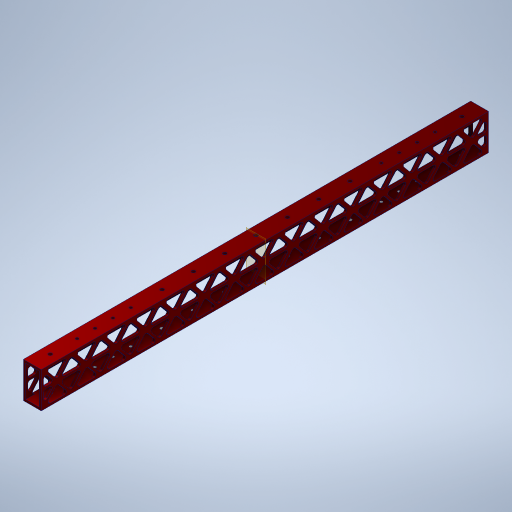
# Autodesk Inventor part: Drivetrain-Front-Back-Extrusions
Saved by Autodesk Inventor 2024.2 (Build 282272000, 272)
## iProperties
Created: 2024-01-04
Part Number: Drivetrain-Front-Back-Extrusions
Material: Aluminum 6061
Document SubType Name: Modeling
Designer: rohan
Density: 2.7 g/cm^3
Appearance: Aluminum - Flat
Author: rohan
Autodesk Inventor part; units mm, degrees
ref_plane "YZ Plane" through (0, 0, 0) normal (1, 0, 0) x (0, 1, 0)
ref_plane "XZ Plane" through (0, 0, 0) normal (0, 1, 0) x (-1, 0, 0)
ref_plane "XY Plane" through (0, 0, 0) normal (0, 0, 1) x (1, 0, 0)
sketch "Sketch1" plane through (0, 0, 0) normal (0, 0, 1) x (1, 0, 0)
  line L0 (-12.7, -25.4) -> (12.7, -25.4)
  line L1 (12.7, -25.4) -> (12.7, 25.4)
  line L2 (12.7, 25.4) -> (-12.7, 25.4)
  line L3 (-12.7, 25.4) -> (-12.7, -25.4)
  line L4 (-12.7, -25.4) -> (12.7, 25.4) construction
  line L5 (12.7, -25.4) -> (-12.7, 25.4) construction
  line L6 (-9.525, -22.225) -> (9.525, -22.225)
  line L7 (9.525, -22.225) -> (9.525, 22.225)
  line L8 (9.525, 22.225) -> (-9.525, 22.225)
  line L9 (-9.525, 22.225) -> (-9.525, -22.225)
  point P0 (0, 0)
  dimension "d0" = 25.4
  dimension "d1" = 50.8
  dimension "d2" = 3.175
  constraints: 20 end point, 4 parallel, 2 midpoint, 2 perpendicular, 1 horizontal, 3 other
  measures "d0" distance of L2.end L1.end
  measures "d1" distance of L1.end L0.end
  measures "d2" distance between parallel lines of L3 L9
extrude "Extrusion1" add sketch "Sketch1" along normal blind 635
sketch "Sketch2" plane through (-12.7, 25.4, 0) normal (0, 1, 0) x (1, 0, 0)
  circle A0 centre (12.7, -25.4) radius 2.5527
  circle A1 centre (12.7, -63.5) radius 2.0193
  line L0 (25.4, 0) -> (25.4, -635) projected
  circle A2 centre (12.7, -88.9) radius 2.0193
  circle A3 centre (12.7, -114.3) radius 2.0193
  circle A4 centre (12.7, -139.7) radius 2.0193
  point P0 (12.7, 0)
  dimension "d5" = 5.1054
  dimension "d6" = 25.4
  dimension "d7" = 4.0386
  dimension "d8" = 63.5
  dimension "d11" = 25.4
  constraints: 5 centre point, 1 vertical, 6 other
  measures "d5" diameter of A0
  measures "d6" distance of A0.centre point (12.7, 0)
  measures "d7" diameter of A1
  measures "d8" distance of A1.centre point (12.7, 0)
  measures "d11" distance of A1.centre A2.centre
extrude "Extrusion2" cut sketch "Sketch2" against normal blind 111.125
ref_plane "Work Plane1" through (0, 0, 317.5) normal (0, 0, 1) x (1, 0, 0)
mirror "Mirror1" about plane through (0, 0, 317.5) normal (0, 0, 1) of "Extrusion2"
sketch "Sketch5" plane through (12.7, -25.4, 0) normal (1, 0, 0) x (0, 0, -1)
  line L0 (-635, 0) -> (-635, 50.8) projected
  line L1 (-635, 25.4) -> (0, 25.4)
  line L2 (0, 50.8) -> (-635, 50.8) projected
  line L3 (-317.5, 50.8) -> (-317.5, 0)
  line L4 (-631.825, 30.1625) -> (-631.825, 37.2672)
  line L5 (-628.65, 26.9875) -> (-622.6851, 26.9875)
  line L6 (-620.2534, 32.204) -> (-626.2184, 39.3087)
  arc A0 (-626.2184, 39.3087) -> (-631.825, 37.2672) centre (-628.65, 37.2672) ccw
  arc A1 (-631.825, 30.1625) -> (-628.65, 26.9875) centre (-628.65, 30.1625) ccw
  arc A2 (-622.6851, 26.9875) -> (-620.2534, 32.204) centre (-622.6851, 30.1625) ccw
  line L7 (-631.825, 20.6375) -> (-631.825, 13.5328)
  line L8 (-628.65, 23.8125) -> (-622.6851, 23.8125)
  line L9 (-620.2534, 18.596) -> (-626.2184, 11.4913)
  arc A3 (-631.825, 13.5328) -> (-626.2184, 11.4913) centre (-628.65, 13.5328) ccw
  arc A4 (-628.65, 23.8125) -> (-631.825, 20.6375) centre (-628.65, 20.6375) ccw
  arc A5 (-620.2534, 18.596) -> (-622.6851, 23.8125) centre (-622.6851, 20.6375) ccw
  line L10 (-626.2184, 11.4913) -> (-620.2534, 18.596)
  line L11 (-617.8218, 16.5545) -> (-623.7867, 9.4497)
  line L12 (-623.7867, 9.4497) -> (-624.6752, 8.3915)
  line L13 (-622.2436, 3.175) -> (-602.7132, 3.175)
  line L14 (-600.2863, 8.3971) -> (-610.0741, 20.0012)
  line L15 (-624.6752, 8.3915) -> (-614.9327, 19.9956)
  arc A6 (-624.6752, 8.3915) -> (-622.2436, 3.175) centre (-622.2436, 6.35) ccw
  arc A7 (-602.7132, 3.175) -> (-600.2863, 8.3971) centre (-602.7132, 6.35) ccw
  arc A8 (-610.0741, 20.0012) -> (-614.9327, 19.9956) centre (-612.5011, 17.9541) ccw
  line L16 (-608.3475, 17.9541) -> (-602.1017, 10.5494)
  line L17 (-604.7305, 18.5904) -> (-599.6748, 12.5965)
  line L18 (-602.3036, 23.8125) -> (-582.8708, 23.8125)
  line L19 (-599.6748, 12.5965) -> (-604.7305, 18.5904)
  line L20 (-604.7305, 18.5904) -> (-595.0141, 7.0711)
  line L21 (-585.4997, 12.5965) -> (-580.4439, 18.5904)
  line L22 (-580.4439, 18.5904) -> (-590.1603, 7.0711)
  arc A9 (-595.0141, 7.0711) -> (-590.1603, 7.0711) centre (-592.5872, 9.1182) ccw
  arc A10 (-602.3036, 23.8125) -> (-604.7305, 18.5904) centre (-602.3036, 20.6375) ccw
  arc A11 (-580.4439, 18.5904) -> (-582.8708, 23.8125) centre (-582.8708, 20.6375) ccw
  line L23 (-623.7867, 41.3503) -> (-615.5957, 41.3503) construction
  line L24 (-622.2436, 47.625) -> (-602.7132, 47.625)
  line L25 (-600.2863, 42.4029) -> (-610.0741, 30.7988)
  line L26 (-624.6752, 42.4085) -> (-614.9327, 30.8044)
  arc A12 (-622.2436, 47.625) -> (-624.6752, 42.4085) centre (-622.2436, 44.45) ccw
  arc A13 (-600.2863, 42.4029) -> (-602.7132, 47.625) centre (-602.7132, 44.45) ccw
  arc A14 (-614.9327, 30.8044) -> (-610.0741, 30.7988) centre (-612.5011, 32.8459) ccw
  line L27 (-608.3475, 32.8459) -> (-602.1017, 40.2506)
  line L28 (-604.7305, 32.2096) -> (-599.6748, 38.2035)
  line L29 (-602.3036, 26.9875) -> (-582.8708, 26.9875)
  line L30 (-599.6748, 38.2035) -> (-604.7305, 32.2096)
  line L31 (-604.7305, 32.2096) -> (-595.0141, 43.7289)
  line L32 (-585.4997, 38.2035) -> (-580.4439, 32.2096)
  line L33 (-580.4439, 32.2096) -> (-590.1603, 43.7289)
  arc A15 (-590.1603, 43.7289) -> (-595.0141, 43.7289) centre (-592.5872, 41.6818) ccw
  arc A16 (-604.7305, 32.2096) -> (-602.3036, 26.9875) centre (-602.3036, 30.1625) ccw
  arc A17 (-582.8708, 26.9875) -> (-580.4439, 32.2096) centre (-582.8708, 30.1625) ccw
  line L34 (-3.175, 30.1625) -> (-3.175, 37.2672)
  line L35 (-6.35, 26.9875) -> (-12.3149, 26.9875)
  line L36 (-14.7466, 32.204) -> (-8.7816, 39.3087)
  arc A18 (-3.175, 37.2672) -> (-8.7816, 39.3087) centre (-6.35, 37.2672) ccw
  arc A19 (-6.35, 26.9875) -> (-3.175, 30.1625) centre (-6.35, 30.1625) ccw
  arc A20 (-14.7466, 32.204) -> (-12.3149, 26.9875) centre (-12.3149, 30.1625) ccw
  arc A21 (-8.7816, 11.4913) -> (-3.175, 13.5328) centre (-6.35, 13.5328) ccw
  line L37 (-3.175, 20.6375) -> (-3.175, 13.5328)
  line L38 (-14.7466, 18.596) -> (-8.7816, 11.4913)
  arc A22 (-3.175, 20.6375) -> (-6.35, 23.8125) centre (-6.35, 20.6375) ccw
  line L39 (-6.35, 23.8125) -> (-12.3149, 23.8125)
  arc A23 (-12.3149, 23.8125) -> (-14.7466, 18.596) centre (-12.3149, 20.6375) ccw
  line L40 (-8.7816, 11.4913) -> (-14.7466, 18.596)
  line L41 (-17.1782, 16.5545) -> (-11.2133, 9.4497)
  line L42 (-11.2133, 9.4497) -> (-10.3248, 8.3915)
  line L43 (-12.7564, 3.175) -> (-32.2868, 3.175)
  line L44 (-34.7137, 8.3971) -> (-24.9259, 20.0012)
  line L45 (-10.3248, 8.3915) -> (-20.0673, 19.9956)
  arc A24 (-12.7564, 3.175) -> (-10.3248, 8.3915) centre (-12.7564, 6.35) ccw
  arc A25 (-34.7137, 8.3971) -> (-32.2868, 3.175) centre (-32.2868, 6.35) ccw
  arc A26 (-20.0673, 19.9956) -> (-24.9259, 20.0012) centre (-22.4989, 17.9541) ccw
  arc A27 (-32.2868, 47.625) -> (-34.7137, 42.4029) centre (-32.2868, 44.45) ccw
  arc A28 (-24.9259, 30.7988) -> (-20.0673, 30.8044) centre (-22.4989, 32.8459) ccw
  line L46 (-12.7564, 47.625) -> (-32.2868, 47.625)
  line L47 (-34.7137, 42.4029) -> (-24.9259, 30.7988)
  line L48 (-11.2133, 41.3503) -> (-19.4043, 41.3503) construction
  line L49 (-10.3248, 42.4085) -> (-20.0673, 30.8044)
  arc A29 (-10.3248, 42.4085) -> (-12.7564, 47.625) centre (-12.7564, 44.45) ccw
  arc A30 (-538.4069, 18.5904) -> (-540.8338, 23.8125) centre (-540.8338, 20.6375) ccw
  arc A31 (-540.8338, 26.9875) -> (-538.4069, 32.2096) centre (-540.8338, 30.1625) ccw
  line L50 (-543.4627, 38.2035) -> (-538.4069, 32.2096)
  line L51 (-538.4069, 32.2096) -> (-548.1233, 43.7289)
  line L52 (-560.2666, 23.8125) -> (-540.8338, 23.8125)
  arc A32 (-558.2493, 42.4029) -> (-560.6762, 47.625) centre (-560.6762, 44.45) ccw
  line L53 (-562.6935, 32.2096) -> (-552.9771, 43.7289)
  line L54 (-562.6935, 32.2096) -> (-557.6378, 38.2035)
  line L55 (-557.6378, 38.2035) -> (-562.6935, 32.2096)
  line L56 (-592.963, 25.4) -> (42.037, 25.4)
  line L57 (-560.2666, 26.9875) -> (-540.8338, 26.9875)
  arc A33 (-568.0371, 20.0012) -> (-572.8957, 19.9956) centre (-570.4641, 17.9541) ccw
  arc A34 (-560.2666, 23.8125) -> (-562.6935, 18.5904) centre (-560.2666, 20.6375) ccw
  line L58 (-575.7848, 16.5545) -> (-581.7497, 9.4497)
  line L59 (-580.2066, 3.175) -> (-560.6762, 3.175)
  line L60 (-582.6382, 8.3915) -> (-572.8957, 19.9956)
  line L61 (-558.2493, 8.3971) -> (-568.0371, 20.0012)
  arc A35 (-560.6762, 3.175) -> (-558.2493, 8.3971) centre (-560.6762, 6.35) ccw
  line L62 (-566.3105, 17.9541) -> (-560.0647, 10.5494)
  line L63 (-562.6935, 18.5904) -> (-557.6378, 12.5965)
  line L64 (-557.6378, 12.5965) -> (-562.6935, 18.5904)
  line L65 (-562.6935, 18.5904) -> (-552.9771, 7.0711)
  line L66 (-543.4627, 12.5965) -> (-538.4069, 18.5904)
  line L67 (-538.4069, 18.5904) -> (-548.1233, 7.0711)
  arc A36 (-552.9771, 7.0711) -> (-548.1233, 7.0711) centre (-550.5502, 9.1182) ccw
  arc A37 (-548.1233, 43.7289) -> (-552.9771, 43.7289) centre (-550.5502, 41.6818) ccw
  line L68 (-582.6382, 42.4085) -> (-572.8957, 30.8044)
  line L69 (-581.7497, 41.3503) -> (-573.5587, 41.3503) construction
  line L70 (-580.2066, 47.625) -> (-560.6762, 47.625)
  arc A38 (-572.8957, 30.8044) -> (-568.0371, 30.7988) centre (-570.4641, 32.8459) ccw
  line L71 (-566.3105, 32.8459) -> (-560.0647, 40.2506)
  arc A39 (-562.6935, 32.2096) -> (-560.2666, 26.9875) centre (-560.2666, 30.1625) ccw
  line L72 (-558.2493, 42.4029) -> (-568.0371, 30.7988)
  arc A40 (-582.6382, 8.3915) -> (-580.2066, 3.175) centre (-580.2066, 6.35) ccw
  arc A41 (-580.2066, 47.625) -> (-582.6382, 42.4085) centre (-580.2066, 44.45) ccw
  arc A42 (-496.3699, 18.5904) -> (-498.7968, 23.8125) centre (-498.7968, 20.6375) ccw
  arc A43 (-498.7968, 26.9875) -> (-496.3699, 32.2096) centre (-498.7968, 30.1625) ccw
  line L73 (-501.4257, 38.2035) -> (-496.3699, 32.2096)
  line L74 (-496.3699, 32.2096) -> (-506.0863, 43.7289)
  line L75 (-518.2296, 23.8125) -> (-498.7968, 23.8125)
  arc A44 (-516.2123, 42.4029) -> (-518.6392, 47.625) centre (-518.6392, 44.45) ccw
  line L76 (-520.6565, 32.2096) -> (-510.9401, 43.7289)
  line L77 (-520.6565, 32.2096) -> (-515.6008, 38.2035)
  line L78 (-515.6008, 38.2035) -> (-520.6565, 32.2096)
  line L79 (-550.926, 25.4) -> (84.074, 25.4)
  line L80 (-518.2296, 26.9875) -> (-498.7968, 26.9875)
  arc A45 (-526.0001, 20.0012) -> (-530.8587, 19.9956) centre (-528.4271, 17.9541) ccw
  arc A46 (-518.2296, 23.8125) -> (-520.6565, 18.5904) centre (-518.2296, 20.6375) ccw
  line L81 (-533.7478, 16.5545) -> (-539.7127, 9.4497)
  line L82 (-538.1696, 3.175) -> (-518.6392, 3.175)
  line L83 (-540.6012, 8.3915) -> (-530.8587, 19.9956)
  line L84 (-516.2123, 8.3971) -> (-526.0001, 20.0012)
  arc A47 (-518.6392, 3.175) -> (-516.2123, 8.3971) centre (-518.6392, 6.35) ccw
  line L85 (-524.2735, 17.9541) -> (-518.0277, 10.5494)
  line L86 (-520.6565, 18.5904) -> (-515.6008, 12.5965)
  line L87 (-515.6008, 12.5965) -> (-520.6565, 18.5904)
  line L88 (-520.6565, 18.5904) -> (-510.9401, 7.0711)
  line L89 (-501.4257, 12.5965) -> (-496.3699, 18.5904)
  line L90 (-496.3699, 18.5904) -> (-506.0863, 7.0711)
  arc A48 (-510.9401, 7.0711) -> (-506.0863, 7.0711) centre (-508.5132, 9.1182) ccw
  arc A49 (-506.0863, 43.7289) -> (-510.9401, 43.7289) centre (-508.5132, 41.6818) ccw
  line L91 (-540.6012, 42.4085) -> (-530.8587, 30.8044)
  line L92 (-539.7127, 41.3503) -> (-531.5217, 41.3503) construction
  line L93 (-538.1696, 47.625) -> (-518.6392, 47.625)
  arc A50 (-530.8587, 30.8044) -> (-526.0001, 30.7988) centre (-528.4271, 32.8459) ccw
  line L94 (-524.2735, 32.8459) -> (-518.0277, 40.2506)
  arc A51 (-520.6565, 32.2096) -> (-518.2296, 26.9875) centre (-518.2296, 30.1625) ccw
  line L95 (-516.2123, 42.4029) -> (-526.0001, 30.7988)
  arc A52 (-540.6012, 8.3915) -> (-538.1696, 3.175) centre (-538.1696, 6.35) ccw
  arc A53 (-538.1696, 47.625) -> (-540.6012, 42.4085) centre (-538.1696, 44.45) ccw
  arc A54 (-454.3329, 18.5904) -> (-456.7598, 23.8125) centre (-456.7598, 20.6375) ccw
  arc A55 (-456.7598, 26.9875) -> (-454.3329, 32.2096) centre (-456.7598, 30.1625) ccw
  line L96 (-459.3887, 38.2035) -> (-454.3329, 32.2096)
  line L97 (-454.3329, 32.2096) -> (-464.0493, 43.7289)
  line L98 (-476.1926, 23.8125) -> (-456.7598, 23.8125)
  arc A56 (-474.1753, 42.4029) -> (-476.6022, 47.625) centre (-476.6022, 44.45) ccw
  line L99 (-478.6195, 32.2096) -> (-468.9031, 43.7289)
  line L100 (-478.6195, 32.2096) -> (-473.5638, 38.2035)
  line L101 (-473.5638, 38.2035) -> (-478.6195, 32.2096)
  line L102 (-508.889, 25.4) -> (126.111, 25.4)
  line L103 (-476.1926, 26.9875) -> (-456.7598, 26.9875)
  arc A57 (-483.9631, 20.0012) -> (-488.8217, 19.9956) centre (-486.3901, 17.9541) ccw
  arc A58 (-476.1926, 23.8125) -> (-478.6195, 18.5904) centre (-476.1926, 20.6375) ccw
  line L104 (-491.7108, 16.5545) -> (-497.6757, 9.4497)
  line L105 (-496.1326, 3.175) -> (-476.6022, 3.175)
  line L106 (-498.5642, 8.3915) -> (-488.8217, 19.9956)
  line L107 (-474.1753, 8.3971) -> (-483.9631, 20.0012)
  arc A59 (-476.6022, 3.175) -> (-474.1753, 8.3971) centre (-476.6022, 6.35) ccw
  line L108 (-482.2365, 17.9541) -> (-475.9907, 10.5494)
  line L109 (-478.6195, 18.5904) -> (-473.5638, 12.5965)
  line L110 (-473.5638, 12.5965) -> (-478.6195, 18.5904)
  line L111 (-478.6195, 18.5904) -> (-468.9031, 7.0711)
  line L112 (-459.3887, 12.5965) -> (-454.3329, 18.5904)
  line L113 (-454.3329, 18.5904) -> (-464.0493, 7.0711)
  arc A60 (-468.9031, 7.0711) -> (-464.0493, 7.0711) centre (-466.4762, 9.1182) ccw
  arc A61 (-464.0493, 43.7289) -> (-468.9031, 43.7289) centre (-466.4762, 41.6818) ccw
  line L114 (-498.5642, 42.4085) -> (-488.8217, 30.8044)
  line L115 (-497.6757, 41.3503) -> (-489.4847, 41.3503) construction
  line L116 (-496.1326, 47.625) -> (-476.6022, 47.625)
  arc A62 (-488.8217, 30.8044) -> (-483.9631, 30.7988) centre (-486.3901, 32.8459) ccw
  line L117 (-482.2365, 32.8459) -> (-475.9907, 40.2506)
  arc A63 (-478.6195, 32.2096) -> (-476.1926, 26.9875) centre (-476.1926, 30.1625) ccw
  line L118 (-474.1753, 42.4029) -> (-483.9631, 30.7988)
  arc A64 (-498.5642, 8.3915) -> (-496.1326, 3.175) centre (-496.1326, 6.35) ccw
  arc A65 (-496.1326, 47.625) -> (-498.5642, 42.4085) centre (-496.1326, 44.45) ccw
  arc A66 (-412.2959, 18.5904) -> (-414.7228, 23.8125) centre (-414.7228, 20.6375) ccw
  arc A67 (-414.7228, 26.9875) -> (-412.2959, 32.2096) centre (-414.7228, 30.1625) ccw
  line L119 (-417.3517, 38.2035) -> (-412.2959, 32.2096)
  line L120 (-412.2959, 32.2096) -> (-422.0123, 43.7289)
  line L121 (-434.1556, 23.8125) -> (-414.7228, 23.8125)
  arc A68 (-432.1383, 42.4029) -> (-434.5652, 47.625) centre (-434.5652, 44.45) ccw
  line L122 (-436.5825, 32.2096) -> (-426.8661, 43.7289)
  line L123 (-436.5825, 32.2096) -> (-431.5268, 38.2035)
  line L124 (-431.5268, 38.2035) -> (-436.5825, 32.2096)
  line L125 (-466.852, 25.4) -> (168.148, 25.4)
  line L126 (-434.1556, 26.9875) -> (-414.7228, 26.9875)
  arc A69 (-441.9261, 20.0012) -> (-446.7847, 19.9956) centre (-444.3531, 17.9541) ccw
  arc A70 (-434.1556, 23.8125) -> (-436.5825, 18.5904) centre (-434.1556, 20.6375) ccw
  line L127 (-449.6738, 16.5545) -> (-455.6387, 9.4497)
  line L128 (-454.0956, 3.175) -> (-434.5652, 3.175)
  line L129 (-456.5272, 8.3915) -> (-446.7847, 19.9956)
  line L130 (-432.1383, 8.3971) -> (-441.9261, 20.0012)
  arc A71 (-434.5652, 3.175) -> (-432.1383, 8.3971) centre (-434.5652, 6.35) ccw
  line L131 (-440.1995, 17.9541) -> (-433.9537, 10.5494)
  line L132 (-436.5825, 18.5904) -> (-431.5268, 12.5965)
  line L133 (-431.5268, 12.5965) -> (-436.5825, 18.5904)
  line L134 (-436.5825, 18.5904) -> (-426.8661, 7.0711)
  line L135 (-417.3517, 12.5965) -> (-412.2959, 18.5904)
  line L136 (-412.2959, 18.5904) -> (-422.0123, 7.0711)
  arc A72 (-426.8661, 7.0711) -> (-422.0123, 7.0711) centre (-424.4392, 9.1182) ccw
  arc A73 (-422.0123, 43.7289) -> (-426.8661, 43.7289) centre (-424.4392, 41.6818) ccw
  line L137 (-456.5272, 42.4085) -> (-446.7847, 30.8044)
  line L138 (-455.6387, 41.3503) -> (-447.4477, 41.3503) construction
  line L139 (-454.0956, 47.625) -> (-434.5652, 47.625)
  arc A74 (-446.7847, 30.8044) -> (-441.9261, 30.7988) centre (-444.3531, 32.8459) ccw
  line L140 (-440.1995, 32.8459) -> (-433.9537, 40.2506)
  arc A75 (-436.5825, 32.2096) -> (-434.1556, 26.9875) centre (-434.1556, 30.1625) ccw
  line L141 (-432.1383, 42.4029) -> (-441.9261, 30.7988)
  arc A76 (-456.5272, 8.3915) -> (-454.0956, 3.175) centre (-454.0956, 6.35) ccw
  arc A77 (-454.0956, 47.625) -> (-456.5272, 42.4085) centre (-454.0956, 44.45) ccw
  arc A78 (-370.2589, 18.5904) -> (-372.6858, 23.8125) centre (-372.6858, 20.6375) ccw
  arc A79 (-372.6858, 26.9875) -> (-370.2589, 32.2096) centre (-372.6858, 30.1625) ccw
  line L142 (-375.3147, 38.2035) -> (-370.2589, 32.2096)
  line L143 (-370.2589, 32.2096) -> (-379.9753, 43.7289)
  line L144 (-392.1186, 23.8125) -> (-372.6858, 23.8125)
  arc A80 (-390.1013, 42.4029) -> (-392.5282, 47.625) centre (-392.5282, 44.45) ccw
  line L145 (-394.5455, 32.2096) -> (-384.8291, 43.7289)
  line L146 (-394.5455, 32.2096) -> (-389.4898, 38.2035)
  line L147 (-389.4898, 38.2035) -> (-394.5455, 32.2096)
  line L148 (-424.815, 25.4) -> (210.185, 25.4)
  line L149 (-392.1186, 26.9875) -> (-372.6858, 26.9875)
  arc A81 (-399.8891, 20.0012) -> (-404.7477, 19.9956) centre (-402.3161, 17.9541) ccw
  arc A82 (-392.1186, 23.8125) -> (-394.5455, 18.5904) centre (-392.1186, 20.6375) ccw
  line L150 (-407.6368, 16.5545) -> (-413.6017, 9.4497)
  line L151 (-412.0586, 3.175) -> (-392.5282, 3.175)
  line L152 (-414.4902, 8.3915) -> (-404.7477, 19.9956)
  line L153 (-390.1013, 8.3971) -> (-399.8891, 20.0012)
  arc A83 (-392.5282, 3.175) -> (-390.1013, 8.3971) centre (-392.5282, 6.35) ccw
  line L154 (-398.1625, 17.9541) -> (-391.9167, 10.5494)
  line L155 (-394.5455, 18.5904) -> (-389.4898, 12.5965)
  line L156 (-389.4898, 12.5965) -> (-394.5455, 18.5904)
  line L157 (-394.5455, 18.5904) -> (-384.8291, 7.0711)
  line L158 (-375.3147, 12.5965) -> (-370.2589, 18.5904)
  line L159 (-370.2589, 18.5904) -> (-379.9753, 7.0711)
  arc A84 (-384.8291, 7.0711) -> (-379.9753, 7.0711) centre (-382.4022, 9.1182) ccw
  arc A85 (-379.9753, 43.7289) -> (-384.8291, 43.7289) centre (-382.4022, 41.6818) ccw
  line L160 (-414.4902, 42.4085) -> (-404.7477, 30.8044)
  line L161 (-413.6017, 41.3503) -> (-405.4107, 41.3503) construction
  line L162 (-412.0586, 47.625) -> (-392.5282, 47.625)
  arc A86 (-404.7477, 30.8044) -> (-399.8891, 30.7988) centre (-402.3161, 32.8459) ccw
  line L163 (-398.1625, 32.8459) -> (-391.9167, 40.2506)
  arc A87 (-394.5455, 32.2096) -> (-392.1186, 26.9875) centre (-392.1186, 30.1625) ccw
  line L164 (-390.1013, 42.4029) -> (-399.8891, 30.7988)
  arc A88 (-414.4902, 8.3915) -> (-412.0586, 3.175) centre (-412.0586, 6.35) ccw
  arc A89 (-412.0586, 47.625) -> (-414.4902, 42.4085) centre (-412.0586, 44.45) ccw
  arc A90 (-328.2219, 18.5904) -> (-330.6488, 23.8125) centre (-330.6488, 20.6375) ccw
  arc A91 (-330.6488, 26.9875) -> (-328.2219, 32.2096) centre (-330.6488, 30.1625) ccw
  line L165 (-333.2777, 38.2035) -> (-328.2219, 32.2096)
  line L166 (-328.2219, 32.2096) -> (-337.9383, 43.7289)
  line L167 (-350.0816, 23.8125) -> (-330.6488, 23.8125)
  arc A92 (-348.0643, 42.4029) -> (-350.4912, 47.625) centre (-350.4912, 44.45) ccw
  line L168 (-352.5085, 32.2096) -> (-342.7921, 43.7289)
  line L169 (-352.5085, 32.2096) -> (-347.4528, 38.2035)
  line L170 (-347.4528, 38.2035) -> (-352.5085, 32.2096)
  line L171 (-382.778, 25.4) -> (252.222, 25.4)
  line L172 (-350.0816, 26.9875) -> (-330.6488, 26.9875)
  arc A93 (-357.8521, 20.0012) -> (-362.7107, 19.9956) centre (-360.2791, 17.9541) ccw
  arc A94 (-350.0816, 23.8125) -> (-352.5085, 18.5904) centre (-350.0816, 20.6375) ccw
  line L173 (-365.5998, 16.5545) -> (-371.5647, 9.4497)
  line L174 (-370.0216, 3.175) -> (-350.4912, 3.175)
  line L175 (-372.4532, 8.3915) -> (-362.7107, 19.9956)
  line L176 (-348.0643, 8.3971) -> (-357.8521, 20.0012)
  arc A95 (-350.4912, 3.175) -> (-348.0643, 8.3971) centre (-350.4912, 6.35) ccw
  line L177 (-356.1255, 17.9541) -> (-349.8797, 10.5494)
  line L178 (-352.5085, 18.5904) -> (-347.4528, 12.5965)
  line L179 (-347.4528, 12.5965) -> (-352.5085, 18.5904)
  line L180 (-352.5085, 18.5904) -> (-342.7921, 7.0711)
  line L181 (-333.2777, 12.5965) -> (-328.2219, 18.5904)
  line L182 (-328.2219, 18.5904) -> (-337.9383, 7.0711)
  arc A96 (-342.7921, 7.0711) -> (-337.9383, 7.0711) centre (-340.3652, 9.1182) ccw
  arc A97 (-337.9383, 43.7289) -> (-342.7921, 43.7289) centre (-340.3652, 41.6818) ccw
  line L183 (-372.4532, 42.4085) -> (-362.7107, 30.8044)
  line L184 (-371.5647, 41.3503) -> (-363.3737, 41.3503) construction
  line L185 (-370.0216, 47.625) -> (-350.4912, 47.625)
  arc A98 (-362.7107, 30.8044) -> (-357.8521, 30.7988) centre (-360.2791, 32.8459) ccw
  line L186 (-356.1255, 32.8459) -> (-349.8797, 40.2506)
  arc A99 (-352.5085, 32.2096) -> (-350.0816, 26.9875) centre (-350.0816, 30.1625) ccw
  line L187 (-348.0643, 42.4029) -> (-357.8521, 30.7988)
  arc A100 (-372.4532, 8.3915) -> (-370.0216, 3.175) centre (-370.0216, 6.35) ccw
  arc A101 (-370.0216, 47.625) -> (-372.4532, 42.4085) centre (-370.0216, 44.45) ccw
  arc A102 (-286.1849, 18.5904) -> (-288.6118, 23.8125) centre (-288.6118, 20.6375) ccw
  arc A103 (-288.6118, 26.9875) -> (-286.1849, 32.2096) centre (-288.6118, 30.1625) ccw
  line L188 (-291.2407, 38.2035) -> (-286.1849, 32.2096)
  line L189 (-286.1849, 32.2096) -> (-295.9013, 43.7289)
  line L190 (-308.0446, 23.8125) -> (-288.6118, 23.8125)
  arc A104 (-306.0273, 42.4029) -> (-308.4542, 47.625) centre (-308.4542, 44.45) ccw
  line L191 (-310.4715, 32.2096) -> (-300.7551, 43.7289)
  line L192 (-310.4715, 32.2096) -> (-305.4158, 38.2035)
  line L193 (-305.4158, 38.2035) -> (-310.4715, 32.2096)
  line L194 (-340.741, 25.4) -> (294.259, 25.4)
  line L195 (-308.0446, 26.9875) -> (-288.6118, 26.9875)
  arc A105 (-315.8151, 20.0012) -> (-320.6737, 19.9956) centre (-318.2421, 17.9541) ccw
  arc A106 (-308.0446, 23.8125) -> (-310.4715, 18.5904) centre (-308.0446, 20.6375) ccw
  line L196 (-323.5628, 16.5545) -> (-329.5277, 9.4497)
  line L197 (-327.9846, 3.175) -> (-308.4542, 3.175)
  line L198 (-330.4162, 8.3915) -> (-320.6737, 19.9956)
  line L199 (-306.0273, 8.3971) -> (-315.8151, 20.0012)
  arc A107 (-308.4542, 3.175) -> (-306.0273, 8.3971) centre (-308.4542, 6.35) ccw
  line L200 (-314.0885, 17.9541) -> (-307.8427, 10.5494)
  line L201 (-310.4715, 18.5904) -> (-305.4158, 12.5965)
  line L202 (-305.4158, 12.5965) -> (-310.4715, 18.5904)
  line L203 (-310.4715, 18.5904) -> (-300.7551, 7.0711)
  line L204 (-291.2407, 12.5965) -> (-286.1849, 18.5904)
  line L205 (-286.1849, 18.5904) -> (-295.9013, 7.0711)
  arc A108 (-300.7551, 7.0711) -> (-295.9013, 7.0711) centre (-298.3282, 9.1182) ccw
  arc A109 (-295.9013, 43.7289) -> (-300.7551, 43.7289) centre (-298.3282, 41.6818) ccw
  line L206 (-330.4162, 42.4085) -> (-320.6737, 30.8044)
  line L207 (-329.5277, 41.3503) -> (-321.3367, 41.3503) construction
  line L208 (-327.9846, 47.625) -> (-308.4542, 47.625)
  arc A110 (-320.6737, 30.8044) -> (-315.8151, 30.7988) centre (-318.2421, 32.8459) ccw
  line L209 (-314.0885, 32.8459) -> (-307.8427, 40.2506)
  arc A111 (-310.4715, 32.2096) -> (-308.0446, 26.9875) centre (-308.0446, 30.1625) ccw
  line L210 (-306.0273, 42.4029) -> (-315.8151, 30.7988)
  arc A112 (-330.4162, 8.3915) -> (-327.9846, 3.175) centre (-327.9846, 6.35) ccw
  arc A113 (-327.9846, 47.625) -> (-330.4162, 42.4085) centre (-327.9846, 44.45) ccw
  arc A114 (-244.1479, 18.5904) -> (-246.5748, 23.8125) centre (-246.5748, 20.6375) ccw
  arc A115 (-246.5748, 26.9875) -> (-244.1479, 32.2096) centre (-246.5748, 30.1625) ccw
  line L211 (-249.2037, 38.2035) -> (-244.1479, 32.2096)
  line L212 (-244.1479, 32.2096) -> (-253.8643, 43.7289)
  line L213 (-266.0076, 23.8125) -> (-246.5748, 23.8125)
  arc A116 (-263.9903, 42.4029) -> (-266.4172, 47.625) centre (-266.4172, 44.45) ccw
  line L214 (-268.4345, 32.2096) -> (-258.7181, 43.7289)
  line L215 (-268.4345, 32.2096) -> (-263.3788, 38.2035)
  line L216 (-263.3788, 38.2035) -> (-268.4345, 32.2096)
  line L217 (-298.704, 25.4) -> (336.296, 25.4)
  line L218 (-266.0076, 26.9875) -> (-246.5748, 26.9875)
  arc A117 (-273.7781, 20.0012) -> (-278.6367, 19.9956) centre (-276.2051, 17.9541) ccw
  arc A118 (-266.0076, 23.8125) -> (-268.4345, 18.5904) centre (-266.0076, 20.6375) ccw
  line L219 (-281.5258, 16.5545) -> (-287.4907, 9.4497)
  line L220 (-285.9476, 3.175) -> (-266.4172, 3.175)
  line L221 (-288.3792, 8.3915) -> (-278.6367, 19.9956)
  line L222 (-263.9903, 8.3971) -> (-273.7781, 20.0012)
  arc A119 (-266.4172, 3.175) -> (-263.9903, 8.3971) centre (-266.4172, 6.35) ccw
  line L223 (-272.0515, 17.9541) -> (-265.8057, 10.5494)
  line L224 (-268.4345, 18.5904) -> (-263.3788, 12.5965)
  line L225 (-263.3788, 12.5965) -> (-268.4345, 18.5904)
  line L226 (-268.4345, 18.5904) -> (-258.7181, 7.0711)
  line L227 (-249.2037, 12.5965) -> (-244.1479, 18.5904)
  line L228 (-244.1479, 18.5904) -> (-253.8643, 7.0711)
  arc A120 (-258.7181, 7.0711) -> (-253.8643, 7.0711) centre (-256.2912, 9.1182) ccw
  arc A121 (-253.8643, 43.7289) -> (-258.7181, 43.7289) centre (-256.2912, 41.6818) ccw
  line L229 (-288.3792, 42.4085) -> (-278.6367, 30.8044)
  line L230 (-287.4907, 41.3503) -> (-279.2997, 41.3503) construction
  line L231 (-285.9476, 47.625) -> (-266.4172, 47.625)
  arc A122 (-278.6367, 30.8044) -> (-273.7781, 30.7988) centre (-276.2051, 32.8459) ccw
  line L232 (-272.0515, 32.8459) -> (-265.8057, 40.2506)
  arc A123 (-268.4345, 32.2096) -> (-266.0076, 26.9875) centre (-266.0076, 30.1625) ccw
  line L233 (-263.9903, 42.4029) -> (-273.7781, 30.7988)
  arc A124 (-288.3792, 8.3915) -> (-285.9476, 3.175) centre (-285.9476, 6.35) ccw
  arc A125 (-285.9476, 47.625) -> (-288.3792, 42.4085) centre (-285.9476, 44.45) ccw
  arc A126 (-202.1109, 18.5904) -> (-204.5378, 23.8125) centre (-204.5378, 20.6375) ccw
  arc A127 (-204.5378, 26.9875) -> (-202.1109, 32.2096) centre (-204.5378, 30.1625) ccw
  line L234 (-207.1667, 38.2035) -> (-202.1109, 32.2096)
  line L235 (-202.1109, 32.2096) -> (-211.8273, 43.7289)
  line L236 (-223.9706, 23.8125) -> (-204.5378, 23.8125)
  arc A128 (-221.9533, 42.4029) -> (-224.3802, 47.625) centre (-224.3802, 44.45) ccw
  line L237 (-226.3975, 32.2096) -> (-216.6811, 43.7289)
  line L238 (-226.3975, 32.2096) -> (-221.3418, 38.2035)
  line L239 (-221.3418, 38.2035) -> (-226.3975, 32.2096)
  line L240 (-256.667, 25.4) -> (378.333, 25.4)
  line L241 (-223.9706, 26.9875) -> (-204.5378, 26.9875)
  arc A129 (-231.7411, 20.0012) -> (-236.5997, 19.9956) centre (-234.1681, 17.9541) ccw
  arc A130 (-223.9706, 23.8125) -> (-226.3975, 18.5904) centre (-223.9706, 20.6375) ccw
  line L242 (-239.4888, 16.5545) -> (-245.4537, 9.4497)
  line L243 (-243.9106, 3.175) -> (-224.3802, 3.175)
  line L244 (-246.3422, 8.3915) -> (-236.5997, 19.9956)
  line L245 (-221.9533, 8.3971) -> (-231.7411, 20.0012)
  arc A131 (-224.3802, 3.175) -> (-221.9533, 8.3971) centre (-224.3802, 6.35) ccw
  line L246 (-230.0145, 17.9541) -> (-223.7687, 10.5494)
  line L247 (-226.3975, 18.5904) -> (-221.3418, 12.5965)
  line L248 (-221.3418, 12.5965) -> (-226.3975, 18.5904)
  line L249 (-226.3975, 18.5904) -> (-216.6811, 7.0711)
  line L250 (-207.1667, 12.5965) -> (-202.1109, 18.5904)
  line L251 (-202.1109, 18.5904) -> (-211.8273, 7.0711)
  arc A132 (-216.6811, 7.0711) -> (-211.8273, 7.0711) centre (-214.2542, 9.1182) ccw
  arc A133 (-211.8273, 43.7289) -> (-216.6811, 43.7289) centre (-214.2542, 41.6818) ccw
  line L252 (-246.3422, 42.4085) -> (-236.5997, 30.8044)
  line L253 (-245.4537, 41.3503) -> (-237.2627, 41.3503) construction
  line L254 (-243.9106, 47.625) -> (-224.3802, 47.625)
  arc A134 (-236.5997, 30.8044) -> (-231.7411, 30.7988) centre (-234.1681, 32.8459) ccw
  line L255 (-230.0145, 32.8459) -> (-223.7687, 40.2506)
  arc A135 (-226.3975, 32.2096) -> (-223.9706, 26.9875) centre (-223.9706, 30.1625) ccw
  line L256 (-221.9533, 42.4029) -> (-231.7411, 30.7988)
  arc A136 (-246.3422, 8.3915) -> (-243.9106, 3.175) centre (-243.9106, 6.35) ccw
  arc A137 (-243.9106, 47.625) -> (-246.3422, 42.4085) centre (-243.9106, 44.45) ccw
  arc A138 (-160.0739, 18.5904) -> (-162.5008, 23.8125) centre (-162.5008, 20.6375) ccw
  arc A139 (-162.5008, 26.9875) -> (-160.0739, 32.2096) centre (-162.5008, 30.1625) ccw
  line L257 (-165.1297, 38.2035) -> (-160.0739, 32.2096)
  line L258 (-160.0739, 32.2096) -> (-169.7903, 43.7289)
  line L259 (-181.9336, 23.8125) -> (-162.5008, 23.8125)
  arc A140 (-179.9163, 42.4029) -> (-182.3432, 47.625) centre (-182.3432, 44.45) ccw
  line L260 (-184.3605, 32.2096) -> (-174.6441, 43.7289)
  line L261 (-184.3605, 32.2096) -> (-179.3048, 38.2035)
  line L262 (-179.3048, 38.2035) -> (-184.3605, 32.2096)
  line L263 (-214.63, 25.4) -> (420.37, 25.4)
  line L264 (-181.9336, 26.9875) -> (-162.5008, 26.9875)
  arc A141 (-189.7041, 20.0012) -> (-194.5627, 19.9956) centre (-192.1311, 17.9541) ccw
  arc A142 (-181.9336, 23.8125) -> (-184.3605, 18.5904) centre (-181.9336, 20.6375) ccw
  line L265 (-197.4518, 16.5545) -> (-203.4167, 9.4497)
  line L266 (-201.8736, 3.175) -> (-182.3432, 3.175)
  line L267 (-204.3052, 8.3915) -> (-194.5627, 19.9956)
  line L268 (-179.9163, 8.3971) -> (-189.7041, 20.0012)
  arc A143 (-182.3432, 3.175) -> (-179.9163, 8.3971) centre (-182.3432, 6.35) ccw
  line L269 (-187.9775, 17.9541) -> (-181.7317, 10.5494)
  line L270 (-184.3605, 18.5904) -> (-179.3048, 12.5965)
  line L271 (-179.3048, 12.5965) -> (-184.3605, 18.5904)
  line L272 (-184.3605, 18.5904) -> (-174.6441, 7.0711)
  line L273 (-165.1297, 12.5965) -> (-160.0739, 18.5904)
  line L274 (-160.0739, 18.5904) -> (-169.7903, 7.0711)
  arc A144 (-174.6441, 7.0711) -> (-169.7903, 7.0711) centre (-172.2172, 9.1182) ccw
  arc A145 (-169.7903, 43.7289) -> (-174.6441, 43.7289) centre (-172.2172, 41.6818) ccw
  line L275 (-204.3052, 42.4085) -> (-194.5627, 30.8044)
  line L276 (-203.4167, 41.3503) -> (-195.2257, 41.3503) construction
  line L277 (-201.8736, 47.625) -> (-182.3432, 47.625)
  arc A146 (-194.5627, 30.8044) -> (-189.7041, 30.7988) centre (-192.1311, 32.8459) ccw
  line L278 (-187.9775, 32.8459) -> (-181.7317, 40.2506)
  arc A147 (-184.3605, 32.2096) -> (-181.9336, 26.9875) centre (-181.9336, 30.1625) ccw
  line L279 (-179.9163, 42.4029) -> (-189.7041, 30.7988)
  arc A148 (-204.3052, 8.3915) -> (-201.8736, 3.175) centre (-201.8736, 6.35) ccw
  arc A149 (-201.8736, 47.625) -> (-204.3052, 42.4085) centre (-201.8736, 44.45) ccw
  arc A150 (-118.0369, 18.5904) -> (-120.4638, 23.8125) centre (-120.4638, 20.6375) ccw
  arc A151 (-120.4638, 26.9875) -> (-118.0369, 32.2096) centre (-120.4638, 30.1625) ccw
  line L280 (-123.0927, 38.2035) -> (-118.0369, 32.2096)
  line L281 (-118.0369, 32.2096) -> (-127.7533, 43.7289)
  line L282 (-139.8966, 23.8125) -> (-120.4638, 23.8125)
  arc A152 (-137.8793, 42.4029) -> (-140.3062, 47.625) centre (-140.3062, 44.45) ccw
  line L283 (-142.3235, 32.2096) -> (-132.6071, 43.7289)
  line L284 (-142.3235, 32.2096) -> (-137.2678, 38.2035)
  line L285 (-137.2678, 38.2035) -> (-142.3235, 32.2096)
  line L286 (-172.593, 25.4) -> (462.407, 25.4)
  line L287 (-139.8966, 26.9875) -> (-120.4638, 26.9875)
  arc A153 (-147.6671, 20.0012) -> (-152.5257, 19.9956) centre (-150.0941, 17.9541) ccw
  arc A154 (-139.8966, 23.8125) -> (-142.3235, 18.5904) centre (-139.8966, 20.6375) ccw
  line L288 (-155.4148, 16.5545) -> (-161.3797, 9.4497)
  line L289 (-159.8366, 3.175) -> (-140.3062, 3.175)
  line L290 (-162.2682, 8.3915) -> (-152.5257, 19.9956)
  line L291 (-137.8793, 8.3971) -> (-147.6671, 20.0012)
  arc A155 (-140.3062, 3.175) -> (-137.8793, 8.3971) centre (-140.3062, 6.35) ccw
  line L292 (-145.9405, 17.9541) -> (-139.6947, 10.5494)
  line L293 (-142.3235, 18.5904) -> (-137.2678, 12.5965)
  line L294 (-137.2678, 12.5965) -> (-142.3235, 18.5904)
  line L295 (-142.3235, 18.5904) -> (-132.6071, 7.0711)
  line L296 (-123.0927, 12.5965) -> (-118.0369, 18.5904)
  line L297 (-118.0369, 18.5904) -> (-127.7533, 7.0711)
  arc A156 (-132.6071, 7.0711) -> (-127.7533, 7.0711) centre (-130.1802, 9.1182) ccw
  arc A157 (-127.7533, 43.7289) -> (-132.6071, 43.7289) centre (-130.1802, 41.6818) ccw
  line L298 (-162.2682, 42.4085) -> (-152.5257, 30.8044)
  line L299 (-161.3797, 41.3503) -> (-153.1887, 41.3503) construction
  line L300 (-159.8366, 47.625) -> (-140.3062, 47.625)
  arc A158 (-152.5257, 30.8044) -> (-147.6671, 30.7988) centre (-150.0941, 32.8459) ccw
  line L301 (-145.9405, 32.8459) -> (-139.6947, 40.2506)
  arc A159 (-142.3235, 32.2096) -> (-139.8966, 26.9875) centre (-139.8966, 30.1625) ccw
  line L302 (-137.8793, 42.4029) -> (-147.6671, 30.7988)
  arc A160 (-162.2682, 8.3915) -> (-159.8366, 3.175) centre (-159.8366, 6.35) ccw
  arc A161 (-159.8366, 47.625) -> (-162.2682, 42.4085) centre (-159.8366, 44.45) ccw
  arc A162 (-75.9999, 18.5904) -> (-78.4268, 23.8125) centre (-78.4268, 20.6375) ccw
  arc A163 (-78.4268, 26.9875) -> (-75.9999, 32.2096) centre (-78.4268, 30.1625) ccw
  line L303 (-81.0557, 38.2035) -> (-75.9999, 32.2096)
  line L304 (-75.9999, 32.2096) -> (-85.7163, 43.7289)
  line L305 (-97.8596, 23.8125) -> (-78.4268, 23.8125)
  arc A164 (-95.8423, 42.4029) -> (-98.2692, 47.625) centre (-98.2692, 44.45) ccw
  line L306 (-100.2865, 32.2096) -> (-90.5701, 43.7289)
  line L307 (-100.2865, 32.2096) -> (-95.2308, 38.2035)
  line L308 (-95.2308, 38.2035) -> (-100.2865, 32.2096)
  line L309 (-130.556, 25.4) -> (504.444, 25.4)
  line L310 (-97.8596, 26.9875) -> (-78.4268, 26.9875)
  arc A165 (-105.6301, 20.0012) -> (-110.4887, 19.9956) centre (-108.0571, 17.9541) ccw
  arc A166 (-97.8596, 23.8125) -> (-100.2865, 18.5904) centre (-97.8596, 20.6375) ccw
  line L311 (-113.3778, 16.5545) -> (-119.3427, 9.4497)
  line L312 (-117.7996, 3.175) -> (-98.2692, 3.175)
  line L313 (-120.2312, 8.3915) -> (-110.4887, 19.9956)
  line L314 (-95.8423, 8.3971) -> (-105.6301, 20.0012)
  arc A167 (-98.2692, 3.175) -> (-95.8423, 8.3971) centre (-98.2692, 6.35) ccw
  line L315 (-103.9035, 17.9541) -> (-97.6577, 10.5494)
  line L316 (-100.2865, 18.5904) -> (-95.2308, 12.5965)
  line L317 (-95.2308, 12.5965) -> (-100.2865, 18.5904)
  line L318 (-100.2865, 18.5904) -> (-90.5701, 7.0711)
  line L319 (-81.0557, 12.5965) -> (-75.9999, 18.5904)
  line L320 (-75.9999, 18.5904) -> (-85.7163, 7.0711)
  arc A168 (-90.5701, 7.0711) -> (-85.7163, 7.0711) centre (-88.1432, 9.1182) ccw
  arc A169 (-85.7163, 43.7289) -> (-90.5701, 43.7289) centre (-88.1432, 41.6818) ccw
  line L321 (-120.2312, 42.4085) -> (-110.4887, 30.8044)
  line L322 (-119.3427, 41.3503) -> (-111.1517, 41.3503) construction
  line L323 (-117.7996, 47.625) -> (-98.2692, 47.625)
  arc A170 (-110.4887, 30.8044) -> (-105.6301, 30.7988) centre (-108.0571, 32.8459) ccw
  line L324 (-103.9035, 32.8459) -> (-97.6577, 40.2506)
  arc A171 (-100.2865, 32.2096) -> (-97.8596, 26.9875) centre (-97.8596, 30.1625) ccw
  line L325 (-95.8423, 42.4029) -> (-105.6301, 30.7988)
  arc A172 (-120.2312, 8.3915) -> (-117.7996, 3.175) centre (-117.7996, 6.35) ccw
  arc A173 (-117.7996, 47.625) -> (-120.2312, 42.4085) centre (-117.7996, 44.45) ccw
  arc A174 (-33.9629, 18.5904) -> (-36.3898, 23.8125) centre (-36.3898, 20.6375) ccw
  arc A175 (-36.3898, 26.9875) -> (-33.9629, 32.2096) centre (-36.3898, 30.1625) ccw
  line L326 (-39.0187, 38.2035) -> (-33.9629, 32.2096)
  line L327 (-33.9629, 32.2096) -> (-43.6793, 43.7289)
  line L328 (-55.8226, 23.8125) -> (-36.3898, 23.8125)
  arc A176 (-53.8053, 42.4029) -> (-56.2322, 47.625) centre (-56.2322, 44.45) ccw
  line L329 (-58.2495, 32.2096) -> (-48.5331, 43.7289)
  line L330 (-58.2495, 32.2096) -> (-53.1938, 38.2035)
  line L331 (-53.1938, 38.2035) -> (-58.2495, 32.2096)
  line L332 (-88.519, 25.4) -> (546.481, 25.4)
  line L333 (-55.8226, 26.9875) -> (-36.3898, 26.9875)
  arc A177 (-63.5931, 20.0012) -> (-68.4517, 19.9956) centre (-66.0201, 17.9541) ccw
  arc A178 (-55.8226, 23.8125) -> (-58.2495, 18.5904) centre (-55.8226, 20.6375) ccw
  line L334 (-71.3408, 16.5545) -> (-77.3057, 9.4497)
  line L335 (-75.7626, 3.175) -> (-56.2322, 3.175)
  line L336 (-78.1942, 8.3915) -> (-68.4517, 19.9956)
  line L337 (-53.8053, 8.3971) -> (-63.5931, 20.0012)
  arc A179 (-56.2322, 3.175) -> (-53.8053, 8.3971) centre (-56.2322, 6.35) ccw
  line L338 (-61.8665, 17.9541) -> (-55.6207, 10.5494)
  line L339 (-58.2495, 18.5904) -> (-53.1938, 12.5965)
  line L340 (-53.1938, 12.5965) -> (-58.2495, 18.5904)
  line L341 (-58.2495, 18.5904) -> (-48.5331, 7.0711)
  line L342 (-39.0187, 12.5965) -> (-33.9629, 18.5904)
  line L343 (-33.9629, 18.5904) -> (-43.6793, 7.0711)
  arc A180 (-48.5331, 7.0711) -> (-43.6793, 7.0711) centre (-46.1062, 9.1182) ccw
  arc A181 (-43.6793, 43.7289) -> (-48.5331, 43.7289) centre (-46.1062, 41.6818) ccw
  line L344 (-78.1942, 42.4085) -> (-68.4517, 30.8044)
  line L345 (-77.3057, 41.3503) -> (-69.1147, 41.3503) construction
  line L346 (-75.7626, 47.625) -> (-56.2322, 47.625)
  arc A182 (-68.4517, 30.8044) -> (-63.5931, 30.7988) centre (-66.0201, 32.8459) ccw
  line L347 (-61.8665, 32.8459) -> (-55.6207, 40.2506)
  arc A183 (-58.2495, 32.2096) -> (-55.8226, 26.9875) centre (-55.8226, 30.1625) ccw
  line L348 (-53.8053, 42.4029) -> (-63.5931, 30.7988)
  arc A184 (-78.1942, 8.3915) -> (-75.7626, 3.175) centre (-75.7626, 6.35) ccw
  arc A185 (-75.7626, 47.625) -> (-78.1942, 42.4085) centre (-75.7626, 44.45) ccw
  point P0 (-631.825, 26.9875)
  point P1 (-631.825, 45.9867)
  point P2 (-615.8738, 26.9875)
  point P3 (-631.825, 23.8125)
  point P4 (-615.8738, 23.8125)
  point P5 (-591.9927, 3.175)
  point P6 (-612.5067, 22.8852)
  point P7 (-605.9205, 20.0012)
  point P8 (-609.1353, 23.8125)
  point P9 (-589.7603, 0.8424)
  point P10 (-595.4141, 0.8424)
  point P11 (-591.9927, 47.625)
  point P12 (-612.5067, 27.9148)
  point P13 (-605.9205, 30.7988)
  point P14 (-609.1353, 26.9875)
  point P15 (-3.175, 26.9875)
  point P16 (-3.175, 45.9867)
  point P17 (-19.1262, 26.9875)
  point P18 (-3.175, 23.8125)
  point P19 (-19.1262, 23.8125)
  point P20 (-22.4933, 22.8852)
  point P21 (-26.6525, 17.9541)
  point P22 (-25.8647, 23.8125)
  point P23 (-22.4933, 27.9148)
  point P24 (-25.8647, 26.9875)
  point P25 (-26.6525, 32.8459)
  point P26 (-549.9557, 47.625)
  point P27 (-567.0983, 23.8125)
  point P28 (-567.0983, 26.9875)
  point P29 (-573.8368, 23.8125)
  point P30 (-570.4697, 22.8852)
  point P31 (-563.8835, 20.0012)
  point P32 (-573.8368, 26.9875)
  point P33 (-549.9557, 3.175)
  point P34 (-570.4697, 27.9148)
  point P35 (-563.8835, 30.7988)
  point P36 (-507.9187, 47.625)
  point P37 (-525.0613, 23.8125)
  point P38 (-525.0613, 26.9875)
  point P39 (-531.7998, 23.8125)
  point P40 (-528.4327, 22.8852)
  point P41 (-521.8465, 20.0012)
  point P42 (-531.7998, 26.9875)
  point P43 (-507.9187, 3.175)
  point P44 (-528.4327, 27.9148)
  point P45 (-521.8465, 30.7988)
  point P46 (-465.8817, 47.625)
  point P47 (-483.0243, 23.8125)
  point P48 (-483.0243, 26.9875)
  point P49 (-489.7628, 23.8125)
  point P50 (-486.3957, 22.8852)
  point P51 (-479.8095, 20.0012)
  point P52 (-489.7628, 26.9875)
  point P53 (-465.8817, 3.175)
  point P54 (-486.3957, 27.9148)
  point P55 (-479.8095, 30.7988)
  point P56 (-423.8447, 47.625)
  point P57 (-440.9873, 23.8125)
  point P58 (-440.9873, 26.9875)
  point P59 (-447.7258, 23.8125)
  point P60 (-444.3587, 22.8852)
  point P61 (-437.7725, 20.0012)
  point P62 (-447.7258, 26.9875)
  point P63 (-423.8447, 3.175)
  point P64 (-444.3587, 27.9148)
  point P65 (-437.7725, 30.7988)
  point P66 (-381.8077, 47.625)
  point P67 (-398.9503, 23.8125)
  point P68 (-398.9503, 26.9875)
  point P69 (-405.6888, 23.8125)
  point P70 (-402.3217, 22.8852)
  point P71 (-395.7355, 20.0012)
  point P72 (-405.6888, 26.9875)
  point P73 (-381.8077, 3.175)
  point P74 (-402.3217, 27.9148)
  point P75 (-395.7355, 30.7988)
  point P76 (-339.7707, 47.625)
  point P77 (-356.9133, 23.8125)
  point P78 (-356.9133, 26.9875)
  point P79 (-363.6518, 23.8125)
  point P80 (-360.2847, 22.8852)
  point P81 (-353.6985, 20.0012)
  point P82 (-363.6518, 26.9875)
  point P83 (-339.7707, 3.175)
  point P84 (-360.2847, 27.9148)
  point P85 (-353.6985, 30.7988)
  point P86 (-297.7337, 47.625)
  point P87 (-314.8763, 23.8125)
  point P88 (-314.8763, 26.9875)
  point P89 (-321.6148, 23.8125)
  point P90 (-318.2477, 22.8852)
  point P91 (-311.6615, 20.0012)
  point P92 (-321.6148, 26.9875)
  point P93 (-297.7337, 3.175)
  point P94 (-318.2477, 27.9148)
  point P95 (-311.6615, 30.7988)
  point P96 (-255.6967, 47.625)
  point P97 (-272.8393, 23.8125)
  point P98 (-272.8393, 26.9875)
  point P99 (-279.5778, 23.8125)
  point P100 (-276.2107, 22.8852)
  point P101 (-269.6245, 20.0012)
  point P102 (-279.5778, 26.9875)
  point P103 (-255.6967, 3.175)
  point P104 (-276.2107, 27.9148)
  point P105 (-269.6245, 30.7988)
  point P106 (-213.6597, 47.625)
  point P107 (-230.8023, 23.8125)
  point P108 (-230.8023, 26.9875)
  point P109 (-237.5408, 23.8125)
  point P110 (-234.1737, 22.8852)
  point P111 (-227.5875, 20.0012)
  point P112 (-237.5408, 26.9875)
  point P113 (-213.6597, 3.175)
  point P114 (-234.1737, 27.9148)
  point P115 (-227.5875, 30.7988)
  point P116 (-171.6227, 47.625)
  point P117 (-188.7653, 23.8125)
  point P118 (-188.7653, 26.9875)
  point P119 (-195.5038, 23.8125)
  point P120 (-192.1367, 22.8852)
  point P121 (-185.5505, 20.0012)
  point P122 (-195.5038, 26.9875)
  point P123 (-171.6227, 3.175)
  point P124 (-192.1367, 27.9148)
  point P125 (-185.5505, 30.7988)
  point P126 (-129.5857, 47.625)
  point P127 (-146.7283, 23.8125)
  point P128 (-146.7283, 26.9875)
  point P129 (-153.4668, 23.8125)
  point P130 (-150.0997, 22.8852)
  point P131 (-143.5135, 20.0012)
  point P132 (-153.4668, 26.9875)
  point P133 (-129.5857, 3.175)
  point P134 (-150.0997, 27.9148)
  point P135 (-143.5135, 30.7988)
  point P136 (-87.5487, 47.625)
  point P137 (-104.6913, 23.8125)
  point P138 (-104.6913, 26.9875)
  point P139 (-111.4298, 23.8125)
  point P140 (-108.0627, 22.8852)
  point P141 (-101.4765, 20.0012)
  point P142 (-111.4298, 26.9875)
  point P143 (-87.5487, 3.175)
  point P144 (-108.0627, 27.9148)
  point P145 (-101.4765, 30.7988)
  point P146 (-45.5117, 47.625)
  point P147 (-62.6543, 23.8125)
  point P148 (-62.6543, 26.9875)
  point P149 (-69.3928, 23.8125)
  point P150 (-66.0257, 22.8852)
  point P151 (-59.4395, 20.0012)
  point P152 (-69.3928, 26.9875)
  point P153 (-45.5117, 3.175)
  point P154 (-66.0257, 27.9148)
  point P155 (-59.4395, 30.7988)
  point P156 (-617.8218, 16.5545)
  point P157 (-575.7848, 16.5545)
  point P158 (-581.7497, 9.4497)
  point P159 (-533.7478, 16.5545)
  point P160 (-539.7127, 9.4497)
  point P161 (-491.7108, 16.5545)
  point P162 (-497.6757, 9.4497)
  point P163 (-449.6738, 16.5545)
  point P164 (-455.6387, 9.4497)
  point P165 (-407.6368, 16.5545)
  point P166 (-413.6017, 9.4497)
  point P167 (-365.5998, 16.5545)
  point P168 (-371.5647, 9.4497)
  point P169 (-239.4888, 16.5545)
  point P170 (-245.4537, 9.4497)
  point P171 (-323.5628, 16.5545)
  point P172 (-329.5277, 9.4497)
  point P173 (-281.5258, 16.5545)
  point P174 (-287.4907, 9.4497)
  point P175 (-197.4518, 16.5545)
  point P176 (-203.4167, 9.4497)
  point P177 (-155.4148, 16.5545)
  point P178 (-161.3797, 9.4497)
  point P179 (-113.3778, 16.5545)
  point P180 (-119.3427, 9.4497)
  point P181 (-17.1782, 16.5545)
  point P182 (-71.3408, 16.5545)
  point P183 (-77.3057, 9.4497)
  dimension "d49" = 18.9992
  dimension "d50" = 3.175
  dimension "d51" = 3.175
  dimension "d52" = 15.9512
  dimension "d53" = 3.175
  dimension "d54" = 3.175
  dimension "d57" = 3.175
  dimension "d58" = 3.175
  dimension "d60" = 3.175
  dimension "d62" = 3.175
  dimension "d65" = 42.037
  constraints: 694 end point, 372 point on circle, 252 point on line, 186 centre point, 89 symmetric about line, 18 tangent, 5 equal radius, 4 horizontal, 2 midpoint, 2 parallel, 2 vertical, 1256 other
  measures "d49" distance of point (-631.825, 26.988) point (-631.825, 45.987)
  measures "d50" horizontal distance of point (-631.825, 26.988) L1
  measures "d51" distance between parallel lines of L0 L4
  measures "d52" distance of point (-631.825, 26.988) point (-615.874, 26.988)
  measures "d53" radius of A0
  measures "d54" distance between parallel lines of L9 L11
  measures "d57" radius of A6
  measures "d58" distance between parallel lines of L16 L17
  measures "d60" diameter of L18 L1
  measures "d62" radius of A10
  measures "d65" distance of L33.start L50.end
extrude "Extrusion5" cut sketch "Sketch5" against normal blind 25.4 contours A105 L199 A107 L197 L3 | L3 L197 A112 L198 L196 A105 | L208 A104 L210 L209 A110 L3 | L3 A110 L206 A113 L208 | L4 A0 L6 A2 L5 A1 | A4 L8 A5 L9 A3 L7 | L15 A8 L14 A7 L13 A6 L12 L11 | A10 L18 A11 L21 L22 A9 L20 L17 | L24 A13 L25 A14 L26 A12 | L28 L31 A15 L33 L32 A17 L29 A16 | A19 L35 A20 L36 A18 L34 | L38 A23 L39 A22 L37 A21 | L41 L42 A24 L43 A25 L44 A26 L45 | L46 A29 L49 A28 L47 A27 | L66 L67 A36 L65 L63 A34 L52 A30 | L57 A39 L53 A37 L51 L50 A31 | L72 L71 A38 L68 A41 L70 A32 | L61 A35 L59 A40 L60 L58 A33 | L89 L90 A48 L88 L86 A46 L75 A42 | L80 A51 L76 A49 L74 L73 A43 | L95 L94 A50 L91 A53 L93 A44 | L84 A47 L82 A52 L83 L81 A45 | L112 L113 A60 L111 L109 A58 L98 A54 | L103 A63 L99 A61 L97 L96 A55 | L118 L117 A62 L114 A65 L116 A56 | L107 A59 L105 A64 L106 L104 A57 | L135 L136 A72 L134 L132 A70 L121 A66 | L126 A75 L122 A73 L120 L119 A67 | L141 L140 A74 L137 A77 L139 A68 | L130 A71 L128 A76 L129 L127 A69 | L158 L159 A84 L157 L155 A82 L144 A78 | L149 A87 L145 A85 L143 L142 A79 | L164 L163 A86 L160 A89 L162 A80 | L153 A83 L151 A88 L152 L150 A81 | L181 L182 A96 L180 L178 A94 L167 A90 | L172 A99 L168 A97 L166 L165 A91 | L187 L186 A98 L183 A101 L185 A92 | L176 A95 L174 A100 L175 L173 A93 | L204 L205 A108 L203 L201 A106 L190 A102 | L195 A111 L191 A109 L189 L188 A103 | L227 L228 A120 L226 L224 A118 L213 A114 | L218 A123 L214 A121 L212 L211 A115 | L233 L232 A122 L229 A125 L231 A116 | L222 A119 L220 A124 L221 L219 A117 | L250 L251 A132 L249 L247 A130 L236 A126 | L241 A135 L237 A133 L235 L234 A127 | L256 L255 A134 L252 A137 L254 A128 | L245 A131 L243 A136 L244 L242 A129 | L273 L274 A144 L272 L270 A142 L259 A138 | L264 A147 L260 A145 L258 L257 A139 | L279 L278 A146 L275 A149 L277 A140 | L268 A143 L266 A148 L267 L265 A141 | L296 L297 A156 L295 L293 A154 L282 A150 | L287 A159 L283 A157 L281 L280 A151 | L302 L301 A158 L298 A161 L300 A152 | L291 A155 L289 A160 L290 L288 A153 | L319 L320 A168 L318 L316 A166 L305 A162 | L310 A171 L306 A169 L304 L303 A163 | L325 L324 A170 L321 A173 L323 A164 | L314 A167 L312 A172 L313 L311 A165 | L342 L343 A180 L341 L339 A178 L328 A174 | L333 A183 L329 A181 L327 L326 A175 | L348 L347 A182 L344 A185 L346 A176 | L337 A179 L335 A184 L336 L334 A177
sketch "Sketch6" plane through (-12.7, 25.4, 0) normal (0, 1, 0) x (1, 0, 0)
  line L0 (0, 0) -> (0, -635) projected
  line L1 (0, -317.5) -> (25.4, -317.5)
  circle A0 centre (12.7, -317.5) radius 2.5527
  line L2 (25.4, 0) -> (25.4, -635) projected
  circle A1 centre (12.7, -361.95) radius 2.5527
  circle A2 centre (12.7, -406.4) radius 2.5527
  circle A3 centre (12.7, -450.85) radius 2.5527
  circle A4 centre (12.7, -273.05) radius 2.5527
  circle A5 centre (12.7, -317.5) radius 2.5527
  circle A6 centre (12.7, -361.95) radius 2.5527
  circle A7 centre (12.7, -406.4) radius 2.5527
  circle A8 centre (12.7, -228.6) radius 2.5527
  circle A9 centre (12.7, -273.05) radius 2.5527
  circle A10 centre (12.7, -317.5) radius 2.5527
  circle A11 centre (12.7, -361.95) radius 2.5527
  circle A12 centre (12.7, -184.15) radius 2.5527
  circle A13 centre (12.7, -228.6) radius 2.5527
  circle A14 centre (12.7, -273.05) radius 2.5527
  circle A15 centre (12.7, -317.5) radius 2.5527
  point P0 (12.7, 0)
  dimension "d72" = 5.1054
  dimension "d75" = 44.45
  dimension "d78" = 44.45
  constraints: 16 centre point, 2 end point, 2 midpoint, 2 vertical, 1 horizontal, 30 other
  measures "d72" diameter of A0
  measures "d75" distance of A0.centre A1.centre
  measures "d78" distance of A0.centre A4.centre
extrude "Extrusion6" cut sketch "Sketch6" against normal blind 127
equation "\"d3\" = Length"
equation "\"Length\" = 635"
body "Solid1"
